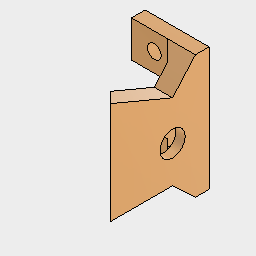
X End Stop Bracket (Autodesk Fusion 360 design; units mm, degrees)
Autodesk Fusion 360 part; units mm, degrees
sketch "Sketch3" plane through (-10.5, 83, -22.5) normal (-1, 0, 0) x (0, -1, 0)
  line L0 (69, 34.5) -> (69, 54.5)
  line L1 (69, 54.5) -> (73, 58.5)
  line L2 (47.5, 56.8252) -> (50.5, 56.8252)
  line L3 (50.5, 56.8252) -> (50.5, 29.8252)
  line L4 (50.5, 29.8252) -> (47.5, 29.8252)
  line L5 (47.5, 29.8252) -> (47.5, 56.8252)
  line L6 (50.5, 48.8252) -> (47.5, 48.8252)
  line L7 (50.5, 37.8252) -> (47.5, 37.8252)
  circle A0 centre (55.5, 42.5) radius 2.75
  line L8 (52.4104, 49.8793) -> (73, 58.5)
  line L9 (73, 58.5) -> (69, 54.5)
  line L10 (69, 54.5) -> (69, 34.5)
  line L11 (69, 34.5) -> (55.5, 34.5)
  arc A1 (52.4104, 49.8793) -> (55.5, 34.5) centre (55.5, 42.5) ccw construction
  circle A2 centre (55.5, 42.5) radius 2.5 construction
  circle A3 centre (55.5, 42.5) radius 8 construction
  line L12 (50.5, 43.3252) -> (47.5, 43.3252) construction
  line L13 (69, 34.5) -> (69, 56.8252)
  line L14 (69, 56.8252) -> (50.5, 56.8252)
  circle A4 centre (55.5, 42.5) radius 6
  line L15 (55.5, 34.5) -> (50.5, 29.8252)
  line L16 (50.5, 56.8252) -> (55.5, 51.1729)
  line L17 (55.5, 34.5) -> (55.5, 51.1729) construction
  dimension "d4250" = 3
  dimension "d4251" = 27
  dimension "d4252" = 11
  dimension "d4253" = 12
  measures "d4250" distance of L2.start L2.end
  measures "d4251" distance of L2.start L4.end
  measures "d4252" distance of L6.end L7.end
  measures "d4253" diameter of A4
extrude "Extrude13" add sketch "Sketch3" along normal blind 4 contours L0 L3 L8 L10 L11 L13 A4 L15 L16 | L3 L4 L5 L7 | L2 L3 L5 L6 | L3 L5 L6 L7 A4
extrude "Extrude14" add sketch "Sketch3" along normal blind 14 contours L3 L4 L5 L7 | L2 L3 L5 L6
extrude "Extrude15" add sketch "Sketch3" along normal blind 2 contours L3 A4 | L3 A4
chamfer "Chamfer11" distance 2 angle 45 2 edges at (-14.5, 32.5, 30.3252) (-14.5, 32.5, 11.3252)
chamfer "Chamfer10" distance 4 angle 45 1 edges at (-14.5, 14, 23.1626)
sketch "Sketch5" plane through (0, 35.5, 0) normal (0, 1, 0) x (-1, 0, 0)
  line L0 (24.5, 34.3252) -> (24.5, 26.3252)
  line L1 (24.5, 15.3252) -> (24.5, 7.3252)
  line L2 (24.5, 34.3252) -> (24.5, 7.3252)
  line L3 (24.5, 20.8252) -> (19.5, 20.8252) construction
  line L4 (19.5, 30.4502) -> (19.5, 11.2002) construction
  dimension "d4263" = 19.25
  dimension "d4264" = 5
  measures "d4263" distance of L4.start L4.end
  measures "d4264" distance of L3.start L3.end
hole "Hole2" at (-19.5, 35.5, 30.4502) at (-19.5, 35.5, 11.2002) direction (0, -1, 0) diameter 3 depth 10 tip angle 118
named bodies: "X End Stop Bracket"
